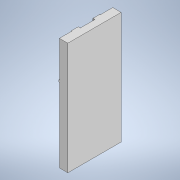
# Autodesk Inventor part: Zplita
Saved by Autodesk Inventor 2020.1 (Build 241239000, 239)
## iProperties
Created: 2023-01-09
Part Number: Zplita
Material: Типовые
Document SubType Name: Modeling
Designer: KirikDK
Density: 1 g/cm^3
Appearance: По умолчанию
Author: KirikDK
Autodesk Inventor part; units mm, degrees
ref_plane "YZ Plane" through (0, 0, 0) normal (1, 0, 0) x (0, 1, 0)
ref_plane "XZ Plane" through (0, 0, 0) normal (0, 1, 0) x (-1, 0, 0)
ref_plane "XY Plane" through (0, 0, 0) normal (0, 0, 1) x (1, 0, 0)
sketch "Эскиз1" plane through (0, 0, 0) normal (0, 1, 0) x (-1, 0, 0)
  line L0 (0, 94.5239) -> (-30, 94.5239)
  line L1 (-30, 94.5239) -> (-30, -95.4761)
  line L2 (-30, -95.4761) -> (0, -95.4761)
  line L3 (0, -95.4761) -> (0, 94.5239)
  line L4 (-30, 50.5239) -> (2, 50.5239)
  line L5 (2, 50.5239) -> (2, -51.4761)
  line L6 (2, -51.4761) -> (-30, -51.4761)
  line L7 (-30, -51.4761) -> (-30, 50.5239)
  point P0 (0, 0)
  point P1 (0, -51.4761)
  point P2 (0, 50.5239)
  dimension "d0" = 190
  dimension "d2" = 30
  dimension "d3" = 32
  dimension "d4" = 44
  dimension "d13" = 44
  constraints: 16 end point, 4 parallel, 2 horizontal, 2 perpendicular, 1 point on line
  measures "d0" distance of L2.end L0.start
  measures "d2" distance of L0.start L0.end
  measures "d3" distance of L4.start L4.end
  measures "d4" distance between parallel lines of L0 L4
  measures "d13" distance between parallel lines of L6 L2
extrude "Выдавливание1" add sketch "Эскиз1" along normal blind 400
sketch "Эскиз2" plane through (-2, 0, -51.4761) normal (-1, 0, 0) x (0, 0, 1)
  line L0 (25, -29) -> (77, -29)
  line L1 (77, -29) -> (77, 456)
  line L2 (77, 456) -> (25, 456)
  line L3 (25, 456) -> (25, -29)
  line L4 (0, 0) -> (102, 0) projected
  line L5 (102, 0) -> (102, 400) projected
  line L6 (0, 400) -> (102, 400) projected
  line L7 (0, 0) -> (0, 400) projected
  point P0 (51.4761, 0)
  point P1 (77, 400)
  point P2 (25, 400)
  point P3 (25, 0)
  point P4 (77, 0)
  dimension "d8" = 25
  dimension "d9" = 25
  dimension "d10" = 52
  constraints: 8 end point, 2 parallel, 1 horizontal, 1 perpendicular
  measures "d8" distance between parallel lines of L7 L3
  measures "d9" distance between parallel lines of L5 L1
  measures "d10" distance of L0.start L0.end
extrude "Выдавливание2" cut sketch "Эскиз2" against normal blind 7.4 contours L3 L6 L1 L4
sketch "Эскиз3" plane through (-2, 0, 50.5239) normal (-1, 0, 0) x (0, 0, 1)
  line L0 (44, 0) -> (44, 400) projected
  line L1 (-146, 0) -> (-146, 400) projected
  line L2 (44, 271.0609) -> (-146, 271.0609)
  line L3 (-146, 271.0609) -> (-146, 264.636)
  line L4 (-146, 264.636) -> (44, 264.636)
  line L5 (44, 264.636) -> (44, 271.0609)
  line L6 (-25, 400) -> (-25, 0) projected
  line L7 (-25, 0) -> (0, 0) projected
  line L8 (0, 0) -> (0, 400) projected
  line L9 (-25, 400) -> (0, 400) projected
  line L10 (-77, 0) -> (-77, 400) projected
  line L11 (-102, 400) -> (-77, 400) projected
  line L12 (-102, 0) -> (-102, 400) projected
  line L13 (-102, 0) -> (-77, 0) projected
  point P0 (-50.5239, 0)
  point P1 (0, 271.0609)
  point P2 (0, 264.636)
  point P3 (-102, 264.636)
  point P4 (-102, 271.0609)
  constraints: 8 end point, 2 parallel, 2 point on line, 1 horizontal, 1 perpendicular
extrude "Выдавливание3" add sketch "Эскиз3" against normal blind 10 contours L4 L8 L2 L0 | L4 L1 L2 L12
